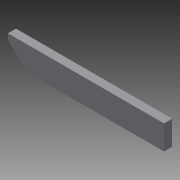
# Autodesk Inventor part: nd-17
Saved by Autodesk Inventor 2015 (Build 190159000, 159)
## iProperties
Created: 2014-07-02
Part Number: nd-17
Material: Generic
Document SubType Name: Modeling
Designer: peter
Density: 1 g/cm^3
Appearance: Default
Author: peter
Autodesk Inventor part; units mm, degrees
ref_plane "YZ Plane" through (0, 0, 0) normal (1, 0, 0) x (0, 1, 0)
ref_plane "XZ Plane" through (0, 0, 0) normal (0, 1, 0) x (-1, 0, 0)
ref_plane "XY Plane" through (0, 0, 0) normal (0, 0, 1) x (1, 0, 0)
sketch "Sketch1" plane through (0, 0, 0) normal (0, 0, 1) x (1, 0, 0)
  line L0 (367.7714, 50.6019) -> (367.7714, -0.1981)
  line L1 (367.7714, -0.1981) -> (367.7714, 56.9519)
  line L2 (367.7714, 56.9519) -> (367.7714, -0.1981)
  line L3 (367.7714, -0.1981) -> (43.93, -0.1981)
  line L4 (43.93, -0.1981) -> (0.2737, 43.4581)
  line L5 (0.2737, 43.4581) -> (0.2737, 56.9519)
  line L6 (0.2737, 56.9519) -> (367.7714, 56.9519)
  point P0 (0, 0)
  constraints: 14 end point, 2 point on line
extrude "Extrusion1" add sketch "Sketch1" along normal blind 19.05
body "Solid1"
